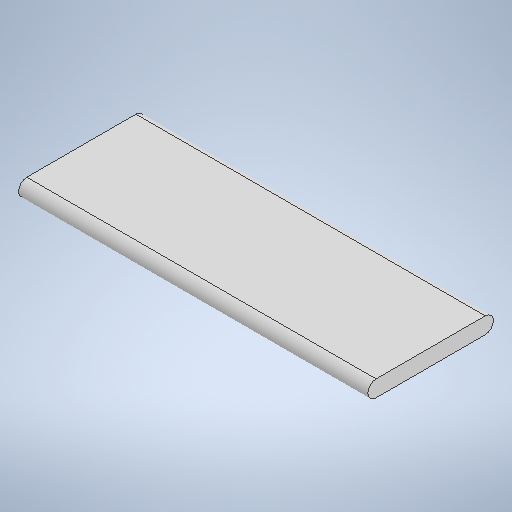
# Autodesk Inventor part: LineupDomioS
Saved by Autodesk Inventor 2025.3 (Build 293356000, 356)
## iProperties
Created: 2025-11-21
Part Number: LineupDomioS
Material: Generic
Document SubType Name: Modeling
Designer: User
Density: 1 g/cm^3
Appearance: Default
Author: User
Autodesk Inventor part; units mm, degrees
ref_plane "YZ Plane" through (0, 0, 0) normal (1, 0, 0) x (0, 1, 0)
ref_plane "XZ Plane" through (0, 0, 0) normal (0, 1, 0) x (-1, 0, 0)
ref_plane "XY Plane" through (0, 0, 0) normal (0, 0, 1) x (1, 0, 0)
sketch "Sketch1" plane through (0, 0, 0) normal (1, 0, 0) x (0, 1, 0)
  line L0 (0, 5) -> (0, -5) construction
  line L1 (-0.75, 5) -> (-0.75, -5)
  line L2 (0.75, -5) -> (0.75, 5)
  arc A0 (0.75, 5) -> (-0.75, 5) centre (0, 5) ccw
  arc A1 (-0.75, -5) -> (0.75, -5) centre (0, -5) ccw
  point P0 (0, 0)
  dimension "d0" = 5
  dimension "d1" = 1.5
  constraints: 8 end point, 4 point on circle, 4 tangent, 2 centre point, 1 midpoint, 1 parallel, 1 vertical
  measures "d0" distance of point (0, 0) L0.end
  measures "d1" diameter of A1
extrude "Extrusion1" add sketch "Sketch1" along normal blind 16 and the other way blind 16
body "Solid1"
